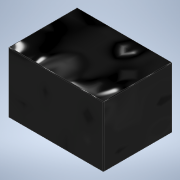
# Autodesk Inventor part: TDN-5_0911
Saved by Autodesk Inventor 2020 (Build 240168000, 168)
## iProperties
Created: 2020-03-12
Part Number: TDN-5_0911
Material: Generisch
Document SubType Name: Modeling
Designer: Marcel-Laptop
Density: 1 g/cm^3
Appearance: Schwarz
Author: Marcel-Laptop
Autodesk Inventor part; units mm, degrees
ref_plane "YZ Plane" through (0, 0, 0) normal (1, 0, 0) x (0, 1, 0)
ref_plane "XZ Plane" through (0, 0, 0) normal (0, 1, 0) x (-1, 0, 0)
ref_plane "XY Plane" through (0, 0, 0) normal (0, 0, 1) x (1, 0, 0)
sketch "Skizze1" plane through (0, 0, 0) normal (0, 0, 1) x (1, 0, 0)
  line L0 (0, 0) -> (14.2, 0)
  line L1 (14.2, 0) -> (14.2, 9.1)
  line L2 (14.2, 9.1) -> (0, 9.1)
  line L3 (0, 9.1) -> (0, 0)
  dimension "d2" = 14.2
  dimension "d3" = 9.1
  constraints: 8 end point, 2 parallel, 1 horizontal, 1 perpendicular
  measures "d2" distance of L1.end L2.end
  measures "d3" distance of L0.end L1.end
extrude "Extrusion1" add sketch "Skizze1" along normal blind 10.2
fillet "Rundung1" radius 0.1 8 edges at (0, 0, 5.1) (0, 4.55, 10.2) (7.1, 9.1, 10.2) (7.1, 0, 10.2) (14.2, 4.55, 10.2) (14.2, 0, 5.1) (14.2, 9.1, 5.1) (0, 9.1, 5.1)
